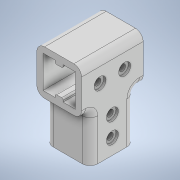
# Autodesk Inventor part: profile_bracket
Saved by Autodesk Inventor 2021 (Build 250183000, 183)
## iProperties
Created: 2021-02-05
Part Number: profile_bracket
Material: 일반
Document SubType Name: Modeling
Designer: jun85
Density: 1 g/cm^3
Appearance: 기본값
Author: jun85
Autodesk Inventor part; units mm, degrees
ref_plane "YZ Plane" through (0, 0, 0) normal (1, 0, 0) x (0, 1, 0)
ref_plane "XZ Plane" through (0, 0, 0) normal (0, 1, 0) x (-1, 0, 0)
sketch "스케치1" plane through (0, 0, 0) normal (0, 0, 1) x (1, 0, 0)
  line L0 (-10.5, -10.5) -> (10.5, -10.5)
  line L1 (10.5, -10.5) -> (10.5, 10.5)
  line L2 (10.5, 10.5) -> (-10.5, 10.5)
  line L3 (-10.5, 10.5) -> (-10.5, -10.5)
  line L4 (-10.5, -10.5) -> (10.5, 10.5) construction
  line L5 (10.5, -10.5) -> (-10.5, 10.5) construction
  line L6 (-2.6, 10.5) -> (2.6, 10.5)
  line L7 (2.6, 10.5) -> (2.6, 8.5)
  line L8 (2.6, 8.5) -> (-2.6, 8.5)
  line L9 (-2.6, 8.5) -> (-2.6, 10.5)
  line L10 (-2.6, -10.5) -> (2.6, -10.5)
  line L11 (2.6, -10.5) -> (2.6, -8.5)
  line L12 (2.6, -8.5) -> (-2.6, -8.5)
  line L13 (-2.6, -8.5) -> (-2.6, -10.5)
  line L14 (0, -20.3) -> (0, 20.3) projected
  line L15 (-14.5, 14.5) -> (14.5, 14.5)
  line L16 (14.5, 14.5) -> (14.5, -14.5)
  line L17 (14.5, -14.5) -> (-14.5, -14.5)
  line L18 (-14.5, -14.5) -> (-14.5, 14.5)
  point P0 (0, 0)
  dimension "d0" = 21
  dimension "d1" = 5.2
  dimension "d2" = 2
  dimension "d3" = 4
  constraints: 36 end point, 8 parallel, 4 perpendicular, 3 equal length, 3 horizontal, 2 midpoint, 2 point on line, 5 other
  measures "d0" distance of L1.end L2.end
  measures "d1" distance of L7.end L8.end
  measures "d2" distance of L6.end L7.end
  measures "d3" distance between parallel lines of L3 L18
extrude "돌출1" add sketch "스케치1" along normal blind 40 contours L0 L14 L17 L18 L15 L2 L3 | L13 L12 L14 L0 | L14 L12 L11 L0 | L0 L1 L2 L14 L15 L16 L17 | L2 L14 L8 L9 | L2 L7 L8 L14
sketch "스케치2" plane through (-14.5, -14.5, 0) normal (0, -1, 0) x (1, 0, 0)
  line L0 (29, 40) -> (0, 40) projected
  line L1 (0, 40) -> (29, 0) construction
  line L2 (29, 0) -> (0, 0) projected
  line L3 (29, 40) -> (0, 0) construction
  line L4 (4, 30.5) -> (25, 30.5)
  line L5 (25, 30.5) -> (25, 9.5)
  line L6 (25, 9.5) -> (4, 9.5)
  line L7 (4, 9.5) -> (4, 30.5)
  line L8 (4, 30.5) -> (25, 9.5) construction
  line L9 (25, 30.5) -> (4, 9.5) construction
  line L10 (29, 5.5) -> (29, 34.5)
  line L11 (29, 34.5) -> (0, 34.5)
  line L12 (0, 34.5) -> (0, 5.5)
  line L13 (0, 5.5) -> (29, 5.5)
  line L14 (11.9, 28.5) -> (17.1, 28.5)
  line L15 (17.1, 28.5) -> (17.1, 30.5)
  line L16 (17.1, 30.5) -> (11.9, 30.5)
  line L17 (11.9, 30.5) -> (11.9, 28.5)
  line L18 (11.9, 28.5) -> (17.1, 30.5) construction
  line L19 (17.1, 28.5) -> (11.9, 30.5) construction
  line L20 (11.9, 9.5) -> (17.1, 9.5)
  line L21 (17.1, 9.5) -> (17.1, 11.5)
  line L22 (17.1, 11.5) -> (11.9, 11.5)
  line L23 (11.9, 11.5) -> (11.9, 9.5)
  line L24 (11.9, 9.5) -> (17.1, 11.5) construction
  line L25 (17.1, 9.5) -> (11.9, 11.5) construction
  point P0 (14.5, 0)
  point P1 (14.5, 20)
  point P2 (14.5, 29.5)
  point P3 (14.5, 10.5)
  point P4 (14.5, 29.5)
  point P5 (14.5, 20)
  point P6 (14.5, 10.5)
  point P7 (14.5, 20)
  point P8 (11.9, 30.5)
  dimension "d6" = 21
  dimension "d7" = 4
  dimension "d8" = 2
  dimension "d9" = 5.2
  constraints: 48 end point, 12 midpoint, 8 parallel, 4 perpendicular, 3 equal length, 3 horizontal, 2 collinear, 2 vertical alignment, 3 other
  measures "d6" distance of L4.end L5.end
  measures "d7" distance between parallel lines of L5 L10
  measures "d8" distance of L14.end L15.end
  measures "d9" distance of L14.start L14.end
extrude "돌출2" add sketch "스케치2" along normal blind 30 contours L4 L15 L14 L17 | L23 L22 L21 L6 | L13 L12 L11 L10
sketch "스케치3" plane through (14.5, -14.5, 0) normal (1, 0, 0) x (0, 0, -1)
  line L0 (0, 25) -> (0, 4) projected
  line L1 (0, 4) -> (-40, 4) projected
  line L2 (-40, 25) -> (-40, 4) projected
  line L3 (0, 25) -> (-40, 25) projected
  line L4 (-9.5, 0) -> (-30.5, 0) projected
  line L5 (-9.5, 0) -> (-9.5, -30) projected
  line L6 (-30.5, -30) -> (-9.5, -30) projected
  line L7 (-30.5, 0) -> (-30.5, -30) projected
  circle A0 centre (-12, 14.5) radius 10.5 construction
  circle A1 centre (-12, 14.5) radius 2.1
  circle A2 centre (-28, 14.5) radius 2.1
  circle A3 centre (-20, -7) radius 10.5 construction
  circle A4 centre (-20, -7) radius 2.1
  circle A5 centre (-20, -20) radius 2.1
  point P0 (0, 14.5)
  dimension "d12" = 4.2
  dimension "d13" = 12
  dimension "d14" = 12
  dimension "d15" = 7
  dimension "d16" = 10
  constraints: 6 centre point, 4 tangent, 3 equal radius, 2 coincident, 1 horizontal alignment, 1 vertical alignment
  measures "d12" diameter of A1
  measures "d13" distance from line of L0 A1.centre
  measures "d14" distance from line of L2 A2.centre
  measures "d15" distance from line of A4.centre L4
  measures "d16" distance from line of L6 A5.centre
extrude "돌출3" cut sketch "스케치3" against normal through all contours A1 | A2 | A4 | A5
sketch "스케치4" plane through (14.5, -14.5, 0) normal (1, 0, 0) x (0, 0, -1)
  circle A0 centre (-28, 14.5) radius 2.1 projected
  circle A1 centre (-12, 14.5) radius 2.1 projected
  line L0 (0, 0) -> (0, 29) projected
  line L1 (0, 29) -> (-40, 29) projected
  line L2 (-40, 0) -> (-40, 29) projected
  line L3 (-34.5, 0) -> (-40, 0) projected
  circle A2 centre (-12, 14.5) radius 3.9
  circle A3 centre (-28, 14.5) radius 3.9
  circle A4 centre (-20, -7) radius 3.9
  circle A5 centre (-20, -20) radius 3.9
  line L4 (-34.5, 0) -> (-34.5, -30) projected
  line L5 (-5.5, -30) -> (-34.5, -30) projected
  line L6 (-5.5, 0) -> (-5.5, -30) projected
  line L7 (0, 0) -> (-5.5, 0) projected
  point P0 (0, 14.5)
  dimension "d19" = 7.8
  constraints: 4 centre point, 3 equal radius, 2 coincident
  measures "d19" diameter of A2
extrude "돌출4" cut sketch "스케치4" against normal blind 1.5 contours A2 | A3 | A4 | A5
ref_plane "작업 평면1" through (0, -10.5, 0) normal (1, 0, 0) x (0, 0, -1)
mirror "미러1" about plane through (0, -10.5, 0) normal (1, 0, 0) of "돌출4"
fillet "모깎기1" radius 5 10 edges at (14.5, -14.5, 2.75) (14.5, -29.5, 5.5) (-14.5, -14.5, 2.75) (-14.5, -29.5, 5.5) (14.5, -14.5, 37.25) (-14.5, -14.5, 37.25) (-14.5, -29.5, 34.5) (14.5, -29.5, 34.5) (14.5, 14.5, 20) (-14.5, 14.5, 20)
fillet "모깎기1" radius 3 2 edges at (0, -14.5, 34.5) (0, -14.5, 5.5)
fillet "모깎기1" radius 1 8 edges at (2.6, 8.5, 20) (-2.6, 8.5, 20) (2.6, -8.5, 20) (-2.6, -8.5, 20) (2.6, -29.5, 11.5) (-2.6, -29.5, 11.5) (-2.6, -29.5, 28.5) (2.6, -29.5, 28.5)
sketch "스케치5" plane through (2.6, -14.5, 30.5) normal (0, -1, 0) x (1, 0, 0)
  line L0 (7.9, 0) -> (0, 0) projected
  line L1 (0, 0) -> (0, -1) projected
  arc A0 (-1, -2) -> (0, -1) centre (-1, -1) ccw projected
  line L2 (-1, -2) -> (-4.2, -2) projected
  arc A1 (-5.2, -1) -> (-4.2, -2) centre (-4.2, -1) ccw projected
  line L3 (-5.2, -1) -> (-5.2, 0) projected
  line L4 (-5.2, 0) -> (-13.1, 0) projected
  line L5 (-13.1, 0) -> (-13.1, -21) projected
  line L6 (-13.1, -21) -> (-5.2, -21) projected
  line L7 (-5.2, -21) -> (-5.2, -20) projected
  arc A2 (-4.2, -19) -> (-5.2, -20) centre (-4.2, -20) ccw projected
  line L8 (-4.2, -19) -> (-1, -19) projected
  arc A3 (0, -20) -> (-1, -19) centre (-1, -20) ccw projected
  line L9 (0, -20) -> (0, -21) projected
  line L10 (0, -21) -> (7.9, -21) projected
  line L11 (7.9, -21) -> (7.9, 0) projected
  line L12 (-10.6, -18.5) -> (-10.6, -2.5)
  line L13 (-10.6, -2.5) -> (-7.3623, -2.5)
  arc A4 (-7.3623, -2.5) -> (-4.2, -4.5) centre (-4.2, -1) ccw
  line L14 (-4.2, -4.5) -> (-1, -4.5)
  arc A5 (-1, -4.5) -> (2.1623, -2.5) centre (-1, -1) ccw
  line L15 (2.1623, -2.5) -> (5.4, -2.5)
  line L16 (5.4, -2.5) -> (5.4, -18.5)
  line L17 (5.4, -18.5) -> (2.1623, -18.5)
  arc A6 (2.1623, -18.5) -> (-1, -16.5) centre (-1, -20) ccw
  line L18 (-1, -16.5) -> (-4.2, -16.5)
  arc A7 (-4.2, -16.5) -> (-7.3623, -18.5) centre (-4.2, -20) ccw
  line L19 (-7.3623, -18.5) -> (-10.6, -18.5)
  point P0 (-2.6, -30.5)
  dimension "d25" = 2.5
  constraints: 16 end point, 8 point on circle, 4 centre point, 11 other
  measures "d25" distance between parallel lines of L12 L5
extrude "돌출5" cut sketch "스케치5" against normal blind 2 contours L11 L10 L9 A3 L8 A2 L7 L6 L5 L4 L3 A1 L2 A0 L1 L0 | L12 L13 A4 L14 A5 L15 L16 L17 A6 L18 A7 L19
